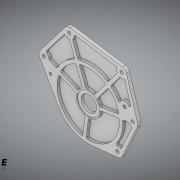
# Autodesk Inventor part: 後ろ脚内フレーム２
Saved by Autodesk Inventor 2020 (Build 240168000, 168)
## iProperties
Created: 2019-09-18
Part Number: 後ろ脚内フレーム２
Material: アルミニウム 2014-T4
Document SubType Name: Modeling
Designer: tanjihayato
Density: 2.8 g/cm^3
Appearance: サテン
Mass: 21.8846 g
Surface Area: 133.053 cm^2
Volume: 7.81591 cm^3
Author: tanjihayato
Autodesk Inventor part; units mm, degrees
ref_plane "YZ Plane" through (0, 0, 0) normal (1, 0, 0) x (0, 1, 0)
ref_plane "XZ Plane" through (0, 0, 0) normal (0, 1, 0) x (-1, 0, 0)
sketch "スケッチ1" plane through (0, 0, 0) normal (0, 0, 1) x (1, 0, 0)
  circle A0 centre (-21.6908, -16.4118) radius 19.1 construction
  circle A1 centre (-58.0056, -24.4791) radius 22.1 construction
  circle A2 centre (-105.5257, -16.4118) radius 30.1 construction
  circle A3 centre (-122.6945, 30.2622) radius 1.5
  circle A4 centre (-75.5257, 23.124) radius 1.5
  circle A5 centre (-65.5257, -10.4118) radius 1.5
  circle A6 centre (-145.5257, 0.5882) radius 1.5
  circle A7 centre (-105.5257, -16.4118) radius 7.025
  circle A8 centre (-21.6908, -16.4118) radius 1.5
  arc A9 (-17.8785, -18.8026) -> (-19.2493, -12.6317) centre (-21.6908, -16.4118) ccw
  arc A10 (-61.0009, -47.384) -> (-50.9717, -46.4821) centre (-58.0056, -24.4791) ccw
  circle A11 centre (-34.2292, -36.4056) radius 1.5
  circle A12 centre (-41.5152, -3.6073) radius 1.5
  arc A13 (-39.0737, 0.1727) -> (-41.3386, 0.8892) centre (-41.5152, -3.6073) ccw
  arc A14 (-32.8589, -40.6919) -> (-30.4168, -38.7963) centre (-34.2292, -36.4056) ccw
  circle A15 centre (-79.2726, -40.4563) radius 1.5
  arc A16 (-78.813, -44.9328) -> (-75.1806, -42.3286) centre (-79.2726, -40.4563) ccw
  line L0 (-17.8785, -18.8026) -> (-30.4168, -38.7963)
  line L1 (-32.8589, -40.6919) -> (-50.9717, -46.4821)
  line L2 (-19.2493, -12.6317) -> (-39.0737, 0.1727)
  arc A17 (-149.0922, 3.3323) -> (-149.4523, -1.6098) centre (-145.5257, 0.5882) ccw
  line L3 (-149.4523, -1.6098) -> (-132.6633, -31.6026)
  line L4 (-102.3494, -47.3492) -> (-78.813, -44.9328)
  line L5 (-61.0009, -47.384) -> (-79.8561, -44.9183)
  circle A18 centre (-72.8083, -2.3784) radius 1.5
  arc A19 (-72.6317, 2.1181) -> (-76.944, -4.1523) centre (-72.8083, -2.3784) ccw
  line L6 (-41.3386, 0.8892) -> (-72.6317, 2.1181)
  arc A20 (-61.4337, -12.2841) -> (-61.2133, -9.1259) centre (-65.5257, -10.4118) ccw
  line L7 (-61.4337, -12.2841) -> (-75.1806, -42.3286)
  arc A21 (-82.5911, -37.417) -> (-76.944, -4.1523) centre (-105.5257, -16.4118) ccw
  arc A22 (-132.6633, -31.6026) -> (-102.3494, -47.3492) centre (-105.5257, -16.4118) ccw
  arc A23 (-122.0212, 34.7115) -> (-126.261, 33.0062) centre (-122.6945, 30.2622) ccw
  arc A24 (-71.2133, 24.4099) -> (-74.8523, 27.5733) centre (-75.5257, 23.124) ccw
  line L8 (-126.261, 33.0062) -> (-149.0922, 3.3323)
  line L9 (-122.0212, 34.7115) -> (-74.8523, 27.5733)
  line L10 (-71.2133, 24.4099) -> (-61.2133, -9.1259)
  circle A25 centre (-58.0056, -24.4791) radius 1.5
  point P0 (0, 0)
  point P1 (0, 0)
  dimension "d0" = 14.05
  dimension "d1" = 3
  dimension "d2" = 3
  dimension "d3" = 1
  dimension "d4" = 3
  dimension "d5" = 3
  dimension "d6" = 3
  dimension "d7" = 3
  dimension "d8" = 3
  dimension "d9" = 3
  dimension "d10" = 9
  dimension "d11" = 3
  dimension "d12" = 3
  dimension "d13" = 9
  dimension "d14" = 31.1
  dimension "d15" = 31.1
  dimension "d16" = 9
  dimension "d17" = 9
  dimension "d18" = 3
  constraints: 30 tangent, 26 centre point, 24 point on circle, 22 end point, 9 coincident
  measures "d0" diameter of A7
  measures "d1" diameter of A8
  measures "d2" radial gap between concentric circles of A8 A9
  measures "d3" radial gap between concentric circles of A1 A10
  measures "d4" diameter of A11
  measures "d5" diameter of A12
  measures "d6" radial gap between concentric circles of A12 A13
  measures "d7" radial gap between concentric circles of A11 A14
  measures "d8" diameter of A15
  measures "d9" radial gap between concentric circles of A15 A16
  measures "d10" diameter of A17
  measures "d11" diameter of A18
  measures "d12" radial gap between concentric circles of A18 A19
  measures "d13" diameter of A20
  measures "d14" radius of A22
  measures "d15" radius of A21
  measures "d16" diameter of A23
  measures "d17" diameter of A24
  measures "d18" diameter of A25
extrude "押し出し1" add sketch "スケッチ1" along normal blind 3 contours L10 A20 L7 A16 L4 A22 L3 A17 L8 A23 L9 A24
sketch "スケッチ2" plane through (0, 0, 3) normal (0, 0, 1) x (1, 0, 0)
  circle A0 centre (-105.5257, -16.4118) radius 30.1 construction
  line L0 (-132.6633, -31.6026) -> (-149.4523, -1.6098) projected
  circle A1 centre (-139.5445, -10.0968) radius 4.5 construction
  line L1 (-149.4523, -1.6098) -> (-132.6633, -31.6026) projected
  circle A2 centre (-139.5445, -10.0968) radius 1.25
  point P0 (0, 0)
  dimension "d21" = 9
  dimension "d22" = 2.5
  constraints: 2 centre point, 2 tangent, 1 coincident
  measures "d21" diameter of A1
  measures "d22" diameter of A2
extrude "押し出し2" cut sketch "スケッチ2" against normal blind 10
sketch "スケッチ3" plane through (0, 0, 3) normal (0, 0, 1) x (1, 0, 0)
  circle A0 centre (-139.5445, -10.0968) radius 1.25 projected
  circle A1 centre (-105.5257, -16.4118) radius 7.025 projected
  circle A2 centre (-72.8083, -2.3784) radius 1.5 projected
  circle A3 centre (-79.2726, -40.4563) radius 1.5 projected
  circle A4 centre (-145.5257, 0.5882) radius 1.5 projected
  circle A5 centre (-65.5257, -10.4118) radius 1.5 projected
  circle A6 centre (-75.5257, 23.124) radius 1.5 projected
  circle A7 centre (-122.6945, 30.2622) radius 1.5 projected
  line L0 (-126.261, 33.0062) -> (-149.0922, 3.3323) projected
  arc A8 (-149.0922, 3.3323) -> (-149.4523, -1.6098) centre (-145.5257, 0.5882) ccw projected
  line L1 (-149.4523, -1.6098) -> (-132.6633, -31.6026) projected
  arc A9 (-132.6633, -31.6026) -> (-102.3494, -47.3492) centre (-105.5257, -16.4118) ccw projected
  line L2 (-102.3494, -47.3492) -> (-78.813, -44.9328) projected
  arc A10 (-78.813, -44.9328) -> (-75.1806, -42.3286) centre (-79.2726, -40.4563) ccw projected
  line L3 (-75.1806, -42.3286) -> (-61.4337, -12.2841) projected
  arc A11 (-61.4337, -12.2841) -> (-61.2133, -9.1259) centre (-65.5257, -10.4118) ccw projected
  line L4 (-61.2133, -9.1259) -> (-71.2133, 24.4099) projected
  arc A12 (-71.2133, 24.4099) -> (-74.8523, 27.5733) centre (-75.5257, 23.124) ccw projected
  line L5 (-74.8523, 27.5733) -> (-122.0212, 34.7115) projected
  arc A13 (-122.0212, 34.7115) -> (-126.261, 33.0062) centre (-122.6945, 30.2622) ccw projected
  line L6 (-118.2752, 31.1105) -> (-79.4961, 25.2419)
  arc A14 (-74.0882, 23.5526) -> (-75.3012, 24.6071) centre (-75.5257, 23.124) ccw
  line L7 (-72.8759, 19.4869) -> (-65.3006, -5.9174)
  arc A15 (-64.1617, -11.0359) -> (-64.0882, -9.9832) centre (-65.5257, -10.4118) ccw
  line L8 (-65.9269, -14.8939) -> (-76.1434, -37.2224)
  arc A16 (-79.1194, -41.9485) -> (-77.9086, -41.0804) centre (-79.2726, -40.4563) ccw
  line L9 (-83.3399, -42.3818) -> (-89.3988, -43.0038)
  arc A17 (-146.7145, 1.5029) -> (-146.8346, -0.1445) centre (-145.5257, 0.5882) ccw
  line L10 (-144.1274, 4.8654) -> (-126.4705, 27.8143)
  arc A18 (-122.47, 31.7453) -> (-123.8833, 31.1769) centre (-122.6945, 30.2622) ccw
  circle A19 centre (-72.8083, -2.3784) radius 4.5
  arc A20 (-76.1434, -37.2224) -> (-82.5911, -37.417) centre (-79.2726, -40.4563) ccw
  circle A21 centre (-105.5257, -16.4118) radius 10.025
  line L11 (-122.6945, 30.2622) -> (-105.5257, -16.4118) construction
  arc A22 (-121.2867, 30.78) -> (-124.1023, 29.7443) centre (-122.6945, 30.2622) ccw
  arc A23 (-106.9334, -16.9296) -> (-104.1179, -15.894) centre (-105.5257, -16.4118) ccw
  line L12 (-75.5257, 23.124) -> (-105.5257, -16.4118) construction
  arc A24 (-74.3307, 22.2173) -> (-76.7206, 24.0307) centre (-75.5257, 23.124) ccw
  arc A25 (-106.7206, -15.5051) -> (-104.3307, -17.3185) centre (-105.5257, -16.4118) ccw
  line L13 (-105.5257, -16.4118) -> (-65.5257, -10.4118) construction
  arc A26 (-105.7482, -14.9284) -> (-105.3032, -17.8952) centre (-105.5257, -16.4118) ccw
  arc A27 (-65.3032, -11.8952) -> (-65.7482, -8.9284) centre (-65.5257, -10.4118) ccw
  line L14 (-145.5257, 0.5882) -> (-105.5257, -16.4118) construction
  arc A28 (-144.939, 1.9687) -> (-146.1124, -0.7923) centre (-145.5257, 0.5882) ccw
  arc A29 (-106.1124, -17.7923) -> (-104.939, -15.0313) centre (-105.5257, -16.4118) ccw
  line L15 (-105.5257, -16.4118) -> (-109.0706, -44.2873) construction
  arc A30 (-104.0377, -16.601) -> (-107.0137, -16.2226) centre (-105.5257, -16.4118) ccw
  arc A31 (-110.298, -45.1495) -> (-107.5826, -44.4765) centre (-109.0706, -44.2873) ccw
  arc A32 (-144.7622, -3.8466) -> (-142.2077, -2.4518) centre (-145.5257, 0.5882) ccw
  arc A33 (-141.0343, 0.3092) -> (-144.1274, 4.8654) centre (-145.5257, 0.5882) ccw
  line L16 (-136.5549, -18.5085) -> (-138.9111, -14.2994)
  line L17 (-142.7957, -7.3597) -> (-144.7622, -3.8466)
  arc A34 (-138.9111, -14.2994) -> (-136.4376, -12.9968) centre (-139.5445, -10.0968) ccw
  arc A35 (-135.6038, -8.5052) -> (-142.7957, -7.3597) centre (-139.5445, -10.0968) ccw
  arc A36 (-136.4376, -12.9968) -> (-136.5549, -18.5085) centre (-105.5257, -16.4118) ccw
  arc A37 (-130.0455, -30.1373) -> (-110.5535, -44.0583) centre (-105.5257, -16.4118) ccw
  arc A38 (-107.5775, -44.4368) -> (-102.6558, -44.3649) centre (-105.5257, -16.4118) ccw
  arc A39 (-132.6633, -31.6026) -> (-102.3494, -47.3492) centre (-105.5257, -16.4118) ccw
  arc A40 (-65.3006, -5.9174) -> (-69.9439, -9.5578) centre (-65.5257, -10.4118) ccw
  arc A41 (-69.4989, -12.5246) -> (-65.9269, -14.8939) centre (-65.5257, -10.4118) ccw
  line L18 (-74.583, -13.2872) -> (-69.4989, -12.5246)
  line L19 (-69.9439, -9.5578) -> (-75.0281, -10.3204)
  line L20 (-85.5533, 7.4275) -> (-76.8953, 18.8375)
  line L21 (-79.2852, 20.6509) -> (-87.9431, 9.241)
  line L22 (-114.842, 13.26) -> (-119.822, 26.7982)
  line L23 (-122.6376, 25.7625) -> (-117.6576, 12.2243)
  line L24 (-133.5279, -2.881) -> (-141.0343, 0.3092)
  line L25 (-142.2077, -2.4518) -> (-134.7014, -5.642)
  arc A42 (-131.9368, -6.8169) -> (-110.5535, -44.0583) centre (-105.5257, -16.4118) ccw
  arc A43 (-134.7014, -5.642) -> (-135.6038, -8.5052) centre (-105.5257, -16.4118) ccw
  arc A44 (-116.6206, 9.4051) -> (-130.7634, -4.0559) centre (-105.5257, -16.4118) ccw
  arc A45 (-117.6576, 12.2243) -> (-133.5279, -2.881) centre (-105.5257, -16.4118) ccw
  arc A46 (-126.4705, 27.8143) -> (-122.6376, 25.7625) centre (-122.6945, 30.2622) ccw
  arc A47 (-119.822, 26.7982) -> (-118.2752, 31.1105) centre (-122.6945, 30.2622) ccw
  arc A48 (-89.7589, 6.848) -> (-113.805, 10.4408) centre (-105.5257, -16.4118) ccw
  arc A49 (-87.9431, 9.241) -> (-114.842, 13.26) centre (-105.5257, -16.4118) ccw
  arc A50 (-79.4961, 25.2419) -> (-79.2852, 20.6509) centre (-75.5257, 23.124) ccw
  arc A51 (-76.8953, 18.8375) -> (-72.8759, 19.4869) centre (-75.5257, 23.124) ccw
  line L26 (-105.3032, -17.8952) -> (-98.5161, -16.8771)
  line L27 (-95.5007, -16.4248) -> (-77.5537, -13.7328)
  line L28 (-77.9987, -10.766) -> (-95.9457, -13.458)
  line L29 (-98.9611, -13.9103) -> (-105.7482, -14.9284)
  line L30 (-104.3307, -17.3185) -> (-100.1822, -11.8513)
  line L31 (-98.339, -9.4223) -> (-87.3691, 5.0346)
  line L32 (-89.7589, 6.848) -> (-100.7289, -7.6089)
  line L33 (-102.5721, -10.0379) -> (-106.7206, -15.5051)
  line L34 (-104.1179, -15.894) -> (-106.4872, -9.4529)
  line L35 (-107.5399, -6.5912) -> (-113.805, 10.4408)
  line L36 (-116.6206, 9.4051) -> (-110.3554, -7.6269)
  line L37 (-109.3028, -10.4886) -> (-106.9334, -16.9296)
  line L38 (-104.939, -15.0313) -> (-111.2552, -12.3469)
  line L39 (-114.0614, -11.1543) -> (-130.7634, -4.0559)
  line L40 (-131.9368, -6.8169) -> (-115.2348, -13.9153)
  line L41 (-112.4286, -15.1079) -> (-106.1124, -17.7923)
  line L42 (-107.0137, -16.2226) -> (-107.8795, -23.0307)
  line L43 (-108.2641, -26.0555) -> (-110.5535, -44.0583)
  line L44 (-107.5775, -44.4368) -> (-105.2881, -26.434)
  line L45 (-104.9034, -23.4092) -> (-104.0377, -16.601)
  arc A52 (-82.5911, -37.417) -> (-74.583, -13.2872) centre (-105.5257, -16.4118) ccw
  arc A53 (-75.0281, -10.3204) -> (-85.5533, 7.4275) centre (-105.5257, -16.4118) ccw
  arc A54 (-107.5775, -44.4368) -> (-77.5537, -13.7328) centre (-105.5257, -16.4118) ccw
  arc A55 (-77.9987, -10.766) -> (-87.3691, 5.0346) centre (-105.5257, -16.4118) ccw
  point P0 (0, 0)
  point P1 (-114.1101, 6.9252)
  point P2 (-90.5257, 3.3561)
  point P3 (-85.5257, -13.4118)
  point P4 (-125.5257, -7.9118)
  point P5 (-107.2981, -30.3496)
  dimension "d28" = 3
  dimension "d25" = 3
  dimension "d27" = 3
  dimension "d30" = 3
  dimension "d31" = 3
  dimension "d32" = 3
  dimension "d33" = 3
  dimension "d38" = 3
  dimension "d39" = 3
  dimension "d40" = 105.778
  dimension "d41" = 105.778
  constraints: 92 end point, 80 point on circle, 56 tangent, 41 centre point, 40 parallel, 5 midpoint, 1 coincident, 1 concentric, 1 point on line, 23 other
  measures "d25" distance between parallel lines of L5 L6
  measures "d27" radial gap between concentric circles of A2 A19
  measures "d30" diameter of A23
  measures "d31" diameter of A25
  measures "d32" diameter of A27
  measures "d33" radial gap between concentric circles of A20 A3
  measures "d38" diameter of A29
  measures "d39" diameter of A31
  measures "d40" angle of L15 L13
  measures "d41" angle of L14 L15
extrude "押し出し3" cut sketch "スケッチ3" against normal blind 2.5 contours L6 A50 L21 A49 L22 A47 | L7 A40 L19 A53 L20 A51 | L8 A20 A52 L18 A41 | L10 A46 L23 A45 L24 A33 | A21 L31 A55 L28 | L27 A54 A38 L44 A21 | A21 L35 A48 L32 | L43 A37 A42 L40 A21 | A21 L39 A44 L36
sketch "スケッチ4" plane through (0, 0, 3) normal (0, 0, 1) x (1, 0, 0)
  arc A0 (-115.2348, -13.9153) -> (-108.2641, -26.0555) centre (-105.5257, -16.4118) ccw projected
  line L0 (-108.2641, -26.0555) -> (-110.5535, -44.0583) projected
  arc A1 (-131.9368, -6.8169) -> (-110.5535, -44.0583) centre (-105.5257, -16.4118) ccw projected
  line L1 (-131.9368, -6.8169) -> (-115.2348, -13.9153) projected
  arc A2 (-119.822, 26.7982) -> (-118.2752, 31.1105) centre (-122.6945, 30.2622) ccw projected
  line L2 (-118.2752, 31.1105) -> (-79.4961, 25.2419) projected
  arc A3 (-79.4961, 25.2419) -> (-79.2852, 20.6509) centre (-75.5257, 23.124) ccw projected
  line L3 (-79.2852, 20.6509) -> (-87.9431, 9.241) projected
  arc A4 (-87.9431, 9.241) -> (-114.842, 13.26) centre (-105.5257, -16.4118) ccw projected
  line L4 (-114.842, 13.26) -> (-119.822, 26.7982) projected
  arc A5 (-76.8953, 18.8375) -> (-72.8759, 19.4869) centre (-75.5257, 23.124) ccw projected
  line L5 (-72.8759, 19.4869) -> (-65.3006, -5.9174) projected
  arc A6 (-65.3006, -5.9174) -> (-69.9439, -9.5578) centre (-65.5257, -10.4118) ccw projected
  line L6 (-69.9439, -9.5578) -> (-75.0281, -10.3204) projected
  arc A7 (-75.0281, -10.3204) -> (-76.944, -4.1523) centre (-105.5257, -16.4118) ccw projected
  arc A8 (-76.944, -4.1523) -> (-85.5533, 7.4275) centre (-105.5257, -16.4118) ccw projected
  line L7 (-85.5533, 7.4275) -> (-76.8953, 18.8375) projected
  line L8 (-114.0614, -11.1543) -> (-130.7634, -4.0559) projected
  arc A9 (-116.6206, 9.4051) -> (-130.7634, -4.0559) centre (-105.5257, -16.4118) ccw projected
  line L9 (-116.6206, 9.4051) -> (-110.3554, -7.6269) projected
  arc A10 (-110.3554, -7.6269) -> (-114.0614, -11.1543) centre (-105.5257, -16.4118) ccw projected
  line L10 (-65.9269, -14.8939) -> (-76.1434, -37.2224) projected
  arc A11 (-76.1434, -37.2224) -> (-82.5911, -37.417) centre (-79.2726, -40.4563) ccw projected
  arc A12 (-82.5911, -37.417) -> (-74.583, -13.2872) centre (-105.5257, -16.4118) ccw projected
  line L11 (-74.583, -13.2872) -> (-69.4989, -12.5246) projected
  arc A13 (-69.4989, -12.5246) -> (-65.9269, -14.8939) centre (-65.5257, -10.4118) ccw projected
  line L12 (-98.339, -9.4223) -> (-87.3691, 5.0346) projected
  arc A14 (-77.9987, -10.766) -> (-87.3691, 5.0346) centre (-105.5257, -16.4118) ccw projected
  line L13 (-77.9987, -10.766) -> (-95.9457, -13.458) projected
  arc A15 (-95.9457, -13.458) -> (-98.339, -9.4223) centre (-105.5257, -16.4118) ccw projected
  arc A16 (-100.7289, -7.6089) -> (-107.5399, -6.5912) centre (-105.5257, -16.4118) ccw projected
  line L14 (-107.5399, -6.5912) -> (-113.805, 10.4408) projected
  arc A17 (-89.7589, 6.848) -> (-113.805, 10.4408) centre (-105.5257, -16.4118) ccw projected
  line L15 (-89.7589, 6.848) -> (-100.7289, -7.6089) projected
  line L16 (-133.5279, -2.881) -> (-141.0343, 0.3092) projected
  arc A18 (-141.0343, 0.3092) -> (-144.1274, 4.8654) centre (-145.5257, 0.5882) ccw projected
  line L17 (-144.1274, 4.8654) -> (-126.4705, 27.8143) projected
  arc A19 (-126.4705, 27.8143) -> (-122.6376, 25.7625) centre (-122.6945, 30.2622) ccw projected
  line L18 (-122.6376, 25.7625) -> (-117.6576, 12.2243) projected
  arc A20 (-117.6576, 12.2243) -> (-133.5279, -2.881) centre (-105.5257, -16.4118) ccw projected
  line L19 (-95.5007, -16.4248) -> (-77.5537, -13.7328) projected
  arc A21 (-107.5775, -44.4368) -> (-77.5537, -13.7328) centre (-105.5257, -16.4118) ccw projected
  line L20 (-107.5775, -44.4368) -> (-105.2881, -26.434) projected
  arc A22 (-105.2881, -26.434) -> (-95.5007, -16.4248) centre (-105.5257, -16.4118) ccw projected
  circle A23 centre (-139.5445, -10.0968) radius 1.25 projected
  circle A24 centre (-105.5257, -16.4118) radius 7.025 projected
  circle A25 centre (-79.2726, -40.4563) radius 1.5 projected
  circle A26 centre (-145.5257, 0.5882) radius 1.5 projected
  circle A27 centre (-65.5257, -10.4118) radius 1.5 projected
  circle A28 centre (-75.5257, 23.124) radius 1.5 projected
  circle A29 centre (-122.6945, 30.2622) radius 1.5 projected
  line L21 (-126.261, 33.0062) -> (-149.0922, 3.3323) projected
  arc A30 (-149.0922, 3.3323) -> (-149.4523, -1.6098) centre (-145.5257, 0.5882) ccw projected
  line L22 (-149.4523, -1.6098) -> (-132.6633, -31.6026) projected
  arc A31 (-132.6633, -31.6026) -> (-102.3494, -47.3492) centre (-105.5257, -16.4118) ccw projected
  line L23 (-102.3494, -47.3492) -> (-78.813, -44.9328) projected
  arc A32 (-78.813, -44.9328) -> (-75.1806, -42.3286) centre (-79.2726, -40.4563) ccw projected
  line L24 (-75.1806, -42.3286) -> (-61.4337, -12.2841) projected
  arc A33 (-61.4337, -12.2841) -> (-61.2133, -9.1259) centre (-65.5257, -10.4118) ccw projected
  line L25 (-61.2133, -9.1259) -> (-71.2133, 24.4099) projected
  arc A34 (-71.2133, 24.4099) -> (-74.8523, 27.5733) centre (-75.5257, 23.124) ccw projected
  line L26 (-74.8523, 27.5733) -> (-122.0212, 34.7115) projected
  arc A35 (-122.0212, 34.7115) -> (-126.261, 33.0062) centre (-122.6945, 30.2622) ccw projected
  circle A36 centre (-105.5257, -16.4118) radius 11
  circle A37 centre (-105.5257, -16.4118) radius 10
  point P0 (0, 0)
  dimension "d44" = 22
  dimension "d45" = 20
  constraints: 2 centre point, 2 coincident
  measures "d44" diameter of A36
  measures "d45" diameter of A37
extrude "押し出し4" add sketch "スケッチ4" against normal blind 2.5 contours L1 A36 L8 A10 L9 L14 A16 L15 L12 A15 L13 L19 A22 L20 L0 A0 | A0 L0 A36 L1 | A36 L9 A10 L8 | L20 A22 L19 A36 | A36 L15 A16 L14 | L13 A15 L12 A36
extrude "押し出し5" cut sketch "スケッチ4" against normal blind 0.5 contours A37
sketch "スケッチ5" plane through (-72.8083, -2.3784, 3) normal (0, 0, 1) x (1, 0, 0)
  arc A0 (3.6342, 2.6538) -> (-4.1186, 1.813) centre (0, 0) ccw
  circle A1 centre (0, 0) radius 1.5 projected
  circle A2 centre (-32.7173, -14.0334) radius 10 projected
  line L0 (-53.4527, 35.3847) -> (-76.2838, 5.7107) projected
  arc A3 (-76.2838, 5.7107) -> (-76.644, 0.7686) centre (-72.7173, 2.9666) ccw projected
  line L1 (-76.644, 0.7686) -> (-59.8549, -29.2242) projected
  arc A4 (-59.8549, -29.2242) -> (-29.5411, -44.9708) centre (-32.7173, -14.0334) ccw projected
  line L2 (-29.5411, -44.9708) -> (-6.0047, -42.5544) projected
  arc A5 (-6.0047, -42.5544) -> (-2.3723, -39.9502) centre (-6.4643, -38.0779) ccw projected
  line L3 (-2.3723, -39.9502) -> (11.3747, -9.9057) projected
  arc A6 (11.3747, -9.9057) -> (11.595, -6.7475) centre (7.2827, -8.0334) ccw projected
  line L4 (11.595, -6.7475) -> (1.595, 26.7883) projected
  arc A7 (1.595, 26.7883) -> (-2.044, 29.9517) centre (-2.7173, 25.5024) ccw projected
  line L5 (-2.044, 29.9517) -> (-49.2128, 37.0899) projected
  arc A8 (-49.2128, 37.0899) -> (-53.4527, 35.3847) centre (-49.8862, 32.6406) ccw projected
  circle A9 centre (-49.8862, 32.6406) radius 1.5 projected
  circle A10 centre (-2.7173, 25.5024) radius 1.5 projected
  circle A11 centre (7.2827, -8.0334) radius 1.5 projected
  circle A12 centre (-72.7173, 2.9666) radius 1.5 projected
  circle A13 centre (-6.4643, -38.0779) radius 1.5 projected
  circle A14 centre (-66.7362, -7.7184) radius 1.25 projected
  line L6 (-60.7196, -0.5026) -> (-68.226, 2.6876) projected
  arc A15 (-68.226, 2.6876) -> (-71.319, 7.2438) centre (-72.7173, 2.9666) ccw projected
  line L7 (-71.319, 7.2438) -> (-53.6621, 30.1927) projected
  arc A16 (-53.6621, 30.1927) -> (-49.8292, 28.1409) centre (-49.8862, 32.6406) ccw projected
  line L8 (-49.8292, 28.1409) -> (-44.8493, 14.6027) projected
  arc A17 (-44.8493, 14.6027) -> (-60.7196, -0.5026) centre (-32.7173, -14.0334) ccw projected
  line L9 (6.8814, -12.5155) -> (-3.3351, -34.844) projected
  arc A18 (-3.3351, -34.844) -> (-9.7828, -35.0386) centre (-6.4643, -38.0779) ccw projected
  arc A19 (-9.7828, -35.0386) -> (-1.7747, -10.9088) centre (-32.7173, -14.0334) ccw projected
  line L10 (-1.7747, -10.9088) -> (3.3095, -10.1461) projected
  arc A20 (3.3095, -10.1461) -> (6.8814, -12.5155) centre (7.2827, -8.0334) ccw projected
  arc A21 (-4.087, 21.2159) -> (-0.0675, 21.8653) centre (-2.7173, 25.5024) ccw projected
  line L11 (-0.0675, 21.8653) -> (7.5078, -3.539) projected
  arc A22 (7.5078, -3.539) -> (2.8645, -7.1793) centre (7.2827, -8.0334) ccw projected
  line L12 (2.8645, -7.1793) -> (-2.2197, -7.942) projected
  arc A23 (-2.2197, -7.942) -> (-4.1356, -1.7739) centre (-32.7173, -14.0334) ccw projected
  arc A24 (-4.1356, -1.7739) -> (-12.7449, 9.8059) centre (-32.7173, -14.0334) ccw projected
  line L13 (-12.7449, 9.8059) -> (-4.087, 21.2159) projected
  arc A25 (-47.0137, 29.1766) -> (-45.4668, 33.4889) centre (-49.8862, 32.6406) ccw projected
  line L14 (-45.4668, 33.4889) -> (-6.6878, 27.6203) projected
  arc A26 (-6.6878, 27.6203) -> (-6.4769, 23.0293) centre (-2.7173, 25.5024) ccw projected
  line L15 (-6.4769, 23.0293) -> (-15.1348, 11.6194) projected
  arc A27 (-15.1348, 11.6194) -> (-42.0337, 15.6384) centre (-32.7173, -14.0334) ccw projected
  line L16 (-42.0337, 15.6384) -> (-47.0137, 29.1766) projected
  arc A28 (-22.1632, -10.9335) -> (-24.9352, -6.2591) centre (-32.7173, -14.0334) ccw projected
  line L17 (-24.9352, -6.2591) -> (-14.5607, 7.413) projected
  arc A29 (-5.1904, -8.3876) -> (-14.5607, 7.413) centre (-32.7173, -14.0334) ccw projected
  line L18 (-5.1904, -8.3876) -> (-22.1632, -10.9335) projected
  line L19 (-35.0716, -3.2883) -> (-40.9967, 12.8192) projected
  arc A30 (-16.9506, 9.2264) -> (-40.9967, 12.8192) centre (-32.7173, -14.0334) ccw projected
  line L20 (-16.9506, 9.2264) -> (-27.3251, -4.4457) projected
  arc A31 (-27.3251, -4.4457) -> (-35.0716, -3.2883) centre (-32.7173, -14.0334) ccw projected
  arc A32 (-32.604, -25.0328) -> (-21.7181, -13.9003) centre (-32.7173, -14.0334) ccw projected
  line L21 (-21.7181, -13.9003) -> (-4.7453, -11.3544) projected
  arc A33 (-34.7692, -42.0584) -> (-4.7453, -11.3544) centre (-32.7173, -14.0334) ccw projected
  line L22 (-34.7692, -42.0584) -> (-32.604, -25.0328) projected
  line L23 (-42.1597, -8.3905) -> (-57.9551, -1.6775) projected
  arc A34 (-43.8122, 11.7835) -> (-57.9551, -1.6775) centre (-32.7173, -14.0334) ccw projected
  line L24 (-43.8122, 11.7835) -> (-37.8872, -4.324) projected
  arc A35 (-37.8872, -4.324) -> (-42.1597, -8.3905) centre (-32.7173, -14.0334) ccw projected
  line L25 (-35.5801, -24.6543) -> (-37.7452, -41.6799) projected
  arc A36 (-59.1285, -4.4385) -> (-37.7452, -41.6799) centre (-32.7173, -14.0334) ccw projected
  line L26 (-59.1285, -4.4385) -> (-43.3331, -11.1515) projected
  arc A37 (-43.3331, -11.1515) -> (-35.5801, -24.6543) centre (-32.7173, -14.0334) ccw projected
  arc A38 (-5.8963, 1.7096) -> (-4.1186, 1.813) centre (-5.0339, 2.2158) ccw
  arc A39 (3.6342, 2.6538) -> (5.4001, 3.5293) centre (4.4418, 3.2436) ccw
  line L27 (-0.0675, 21.8653) -> (7.5078, -3.539) projected
  circle A40 centre (0, 0) radius 4.5 projected
  point P0 (72.8083, 2.3784)
  dimension "d50" = 2
  dimension "d51" = 2
  constraints: 10 point on circle, 4 centre point, 4 tangent, 1 point on line
  measures "d50" diameter of A38
  measures "d51" diameter of A39
extrude "押し出し6" add sketch "スケッチ5" against normal blind 3 contours A39 L11 A22 L12 A23 A40 | A40 A24 A38
fillet "フィレット1" radius 1 40 edges at (-144.1274, 4.8654, 1.75) (-141.0343, 0.3092, 1.75) (-133.5279, -2.881, 1.75) (-130.7634, -4.0559, 1.75) (-131.9368, -6.8169, 1.75) (-116.1415, -13.5299, 1.75) (-114.968, -10.7689, 1.75) (-110.6955, -6.7024, 1.75) (-107.8799, -5.6667, 1.75) (-116.6206, 9.4051, 1.75) (-117.6576, 12.2243, 1.75) (-114.842, 13.26, 1.75) (-113.805, 10.4408, 1.75) (-100.1334, -6.8241, 1.75) (-108.3884, -27.0328, 1.75) (-105.4124, -27.4112, 1.75) (-110.5535, -44.0583, 1.75) (-107.5775, -44.4368, 1.75) (-94.5265, -16.2787, 1.75) (-94.9715, -13.3119, 1.75) (-97.7436, -8.6376, 1.75) (-77.5537, -13.7328, 1.75) (-82.5911, -37.417, 1.75) (-76.1434, -37.2224, 1.75) (-65.9269, -14.8939, 1.75) (-69.4989, -12.5246, 1.75) (-74.583, -13.2872, 1.75) (-77.9987, -10.766, 1.75) (-87.3691, 5.0346, 1.75) (-89.7589, 6.848, 1.75) (-85.5533, 7.4275, 1.75) (-87.9431, 9.241, 1.75) (-72.8759, 19.4869, 1.75) (-76.8953, 18.8375, 1.75) (-79.2852, 20.6509, 1.75) (-79.4961, 25.2419, 1.75) (-119.822, 26.7982, 1.75) (-118.2752, 31.1105, 1.75) (-122.6376, 25.7625, 1.75) (-126.4705, 27.8143, 1.75)
sketch "スケッチ6" plane through (0, 0, 3) normal (0, 0, 1) x (1, 0, 0)
  circle A0 centre (-72.8083, -2.3784) radius 1.5 projected
  circle A1 centre (-105.5257, -16.4118) radius 10 projected
  line L0 (-126.261, 33.0062) -> (-149.0922, 3.3323) projected
  arc A2 (-149.0922, 3.3323) -> (-149.4523, -1.6098) centre (-145.5257, 0.5882) ccw projected
  line L1 (-149.4523, -1.6098) -> (-132.6633, -31.6026) projected
  arc A3 (-132.6633, -31.6026) -> (-102.3494, -47.3492) centre (-105.5257, -16.4118) ccw projected
  line L2 (-102.3494, -47.3492) -> (-78.813, -44.9328) projected
  arc A4 (-78.813, -44.9328) -> (-75.1806, -42.3286) centre (-79.2726, -40.4563) ccw projected
  line L3 (-75.1806, -42.3286) -> (-61.4337, -12.2841) projected
  arc A5 (-61.4337, -12.2841) -> (-61.2133, -9.1259) centre (-65.5257, -10.4118) ccw projected
  line L4 (-61.2133, -9.1259) -> (-71.2133, 24.4099) projected
  arc A6 (-71.2133, 24.4099) -> (-74.8523, 27.5733) centre (-75.5257, 23.124) ccw projected
  line L5 (-74.8523, 27.5733) -> (-122.0212, 34.7115) projected
  arc A7 (-122.0212, 34.7115) -> (-126.261, 33.0062) centre (-122.6945, 30.2622) ccw projected
  circle A8 centre (-122.6945, 30.2622) radius 1.5 projected
  circle A9 centre (-75.5257, 23.124) radius 1.5 projected
  circle A10 centre (-65.5257, -10.4118) radius 1.5 projected
  circle A11 centre (-145.5257, 0.5882) radius 1.5 projected
  circle A12 centre (-79.2726, -40.4563) radius 1.5 projected
  circle A13 centre (-139.5445, -10.0968) radius 1.25 projected
  line L6 (-134.3918, -2.5138) -> (-140.4303, 0.0525) projected
  arc A14 (-141.0367, 0.9029) -> (-140.4303, 0.0525) centre (-140.0391, 0.9728) ccw projected
  arc A15 (-141.0367, 0.9029) -> (-143.1172, 4.3894) centre (-145.5257, 0.5882) ccw projected
  arc A16 (-143.3745, 5.8439) -> (-143.1172, 4.3894) centre (-142.582, 5.2341) ccw projected
  line L7 (-143.3745, 5.8439) -> (-127.2233, 26.8358) projected
  arc A17 (-125.7514, 26.9599) -> (-127.2233, 26.8358) centre (-126.4308, 26.226) ccw projected
  arc A18 (-125.7514, 26.9599) -> (-123.2304, 25.7942) centre (-122.6945, 30.2622) ccw projected
  arc A19 (-122.411, 25.1465) -> (-123.2304, 25.7942) centre (-123.3495, 24.8013) ccw projected
  line L8 (-122.411, 25.1465) -> (-117.9817, 13.1053) projected
  arc A20 (-118.5029, 11.8513) -> (-117.9817, 13.1053) centre (-118.9202, 12.7601) ccw projected
  arc A21 (-118.5029, 11.8513) -> (-133.1136, -2.0551) centre (-105.5257, -16.4118) ccw projected
  arc A22 (-134.3918, -2.5138) -> (-133.1136, -2.0551) centre (-134.0007, -1.5935) ccw projected
  line L9 (-66.4406, -16.0165) -> (-75.6297, -36.0998) projected
  arc A23 (-77.0361, -36.5515) -> (-75.6297, -36.0998) centre (-76.5391, -35.6837) ccw projected
  arc A24 (-77.0361, -36.5515) -> (-79.315, -35.9565) centre (-79.2726, -40.4563) ccw projected
  arc A25 (-80.1407, -34.3788) -> (-79.315, -35.9565) centre (-79.3245, -34.9565) ccw projected
  arc A26 (-80.1407, -34.3788) -> (-74.5039, -14.2077) centre (-105.5257, -16.4118) ccw projected
  arc A27 (-73.6547, -13.1479) -> (-74.5039, -14.2077) centre (-73.5064, -14.1369) ccw projected
  line L10 (-73.6547, -13.1479) -> (-70.1479, -12.6219) projected
  arc A28 (-69.1862, -13.0292) -> (-70.1479, -12.6219) centre (-69.9996, -13.6109) ccw projected
  arc A29 (-69.1862, -13.0292) -> (-67.0182, -14.6571) centre (-65.5257, -10.4118) ccw projected
  arc A30 (-66.4406, -16.0165) -> (-67.0182, -14.6571) centre (-67.3499, -15.6005) ccw projected
  arc A31 (-69.1742, 0.2754) -> (-67.4083, 1.1509) centre (-68.3666, 0.8652) ccw projected
  arc A32 (-69.1742, 0.2754) -> (-76.927, -0.5655) centre (-72.8083, -2.3784) ccw projected
  arc A33 (-78.7046, -0.6688) -> (-76.927, -0.5655) centre (-77.8422, -0.1626) ccw projected
  arc A34 (-78.7046, -0.6688) -> (-84.8539, 6.8237) centre (-105.5257, -16.4118) ccw projected
  arc A35 (-84.9859, 8.1753) -> (-84.8539, 6.8237) centre (-84.1892, 7.5708) ccw projected
  line L11 (-84.9859, 8.1753) -> (-77.2921, 18.3146) projected
  arc A36 (-76.3191, 18.6945) -> (-77.2921, 18.3146) centre (-76.4955, 17.7101) ccw projected
  arc A37 (-76.3191, 18.6945) -> (-73.8531, 18.9464) centre (-75.5257, 23.124) ccw projected
  arc A38 (-72.5231, 18.3038) -> (-73.8531, 18.9464) centre (-73.4814, 18.018) ccw projected
  line L12 (-72.5231, 18.3038) -> (-67.4083, 1.1509) projected
  arc A39 (-119.391, 27.2065) -> (-118.2024, 29.9961) centre (-122.6945, 30.2622) ccw projected
  arc A40 (-117.0545, 30.9257) -> (-118.2024, 29.9961) centre (-117.2041, 29.937) ccw projected
  line L13 (-117.0545, 30.9257) -> (-80.7168, 25.4266) projected
  arc A41 (-79.8954, 24.199) -> (-80.7168, 25.4266) centre (-80.8664, 24.4379) ccw projected
  arc A42 (-79.8954, 24.199) -> (-79.578, 21.1674) centre (-75.5257, 23.124) ccw projected
  arc A43 (-79.6819, 20.1281) -> (-79.578, 21.1674) centre (-80.4786, 20.7325) ccw projected
  line L14 (-79.6819, 20.1281) -> (-87.3757, 9.9888) projected
  arc A44 (-88.7129, 9.752) -> (-87.3757, 9.9888) centre (-88.1723, 10.5932) ccw projected
  arc A45 (-88.7129, 9.752) -> (-113.9565, 13.5236) centre (-105.5257, -16.4118) ccw projected
  arc A46 (-115.1661, 14.141) -> (-113.9565, 13.5236) centre (-114.2276, 14.4862) ccw projected
  line L15 (-115.1661, 14.141) -> (-119.5954, 26.1822) projected
  arc A47 (-119.391, 27.2065) -> (-119.5954, 26.1822) centre (-118.6569, 26.5275) ccw projected
  line L16 (-97.2361, -7.9688) -> (-88.0192, 4.1778) projected
  arc A48 (-86.5472, 4.3108) -> (-88.0192, 4.1778) centre (-87.2226, 3.5733) ccw projected
  arc A49 (-78.2396, -9.6976) -> (-86.5472, 4.3108) centre (-105.5257, -16.4118) ccw projected
  arc A50 (-79.0623, -10.9255) -> (-78.2396, -9.6976) centre (-79.2106, -9.9366) ccw projected
  line L17 (-79.0623, -10.9255) -> (-94.1413, -13.1874) projected
  arc A51 (-95.226, -12.5495) -> (-94.1413, -13.1874) centre (-94.2897, -12.1984) ccw projected
  arc A52 (-95.226, -12.5495) -> (-97.1967, -9.2265) centre (-105.5257, -16.4118) ccw projected
  arc A53 (-97.2361, -7.9688) -> (-97.1967, -9.2265) centre (-96.4395, -8.5733) ccw projected
  line L18 (-108.1697, -4.8789) -> (-113.4337, 9.4314) projected
  arc A54 (-112.7524, 10.743) -> (-113.4337, 9.4314) centre (-112.4952, 9.7767) ccw projected
  arc A55 (-90.6772, 7.4447) -> (-112.7524, 10.743) centre (-105.5257, -16.4118) ccw projected
  arc A56 (-90.409, 5.9913) -> (-90.6772, 7.4447) centre (-91.2057, 6.5957) ccw projected
  line L19 (-90.409, 5.9913) -> (-99.626, -6.1554) projected
  arc A57 (-100.8479, -6.456) -> (-99.626, -6.1554) centre (-100.4226, -5.5509) ccw projected
  arc A58 (-100.8479, -6.456) -> (-107.0891, -5.5235) centre (-105.5257, -16.4118) ccw projected
  arc A59 (-108.1697, -4.8789) -> (-107.0891, -5.5235) centre (-107.2312, -4.5336) ccw projected
  line L20 (-93.6963, -16.1542) -> (-78.6173, -13.8923) projected
  arc A60 (-77.4705, -14.8248) -> (-78.6173, -13.8923) centre (-78.4689, -14.8813) ccw projected
  arc A61 (-106.4839, -44.4955) -> (-77.4705, -14.8248) centre (-105.5257, -16.4118) ccw projected
  arc A62 (-107.4418, -43.3699) -> (-106.4839, -44.4955) centre (-106.4498, -43.496) ccw projected
  line L21 (-107.4418, -43.3699) -> (-105.5183, -28.244) projected
  arc A63 (-104.6095, -27.3736) -> (-105.5183, -28.244) centre (-104.5263, -28.3701) ccw projected
  arc A64 (-104.6095, -27.3736) -> (-94.5461, -17.0822) centre (-105.5257, -16.4118) ccw projected
  arc A65 (-93.6963, -16.1542) -> (-94.5461, -17.0822) centre (-93.548, -17.1431) ccw projected
  line L22 (-115.7406, -10.4406) -> (-129.7736, -4.4766) projected
  arc A66 (-130.2628, -3.0819) -> (-129.7736, -4.4766) centre (-129.3824, -3.5563) ccw projected
  arc A67 (-117.6181, 8.9532) -> (-130.2628, -3.0819) centre (-105.5257, -16.4118) ccw projected
  arc A68 (-116.2493, 8.3957) -> (-117.6181, 8.9532) centre (-117.1878, 8.0505) ccw projected
  line L23 (-116.2493, 8.3957) -> (-110.9853, -5.9145) projected
  arc A69 (-111.3906, -7.1058) -> (-110.9853, -5.9145) centre (-111.9238, -6.2598) ccw projected
  arc A70 (-111.3906, -7.1058) -> (-114.5308, -10.0946) centre (-105.5257, -16.4118) ccw projected
  arc A71 (-115.7406, -10.4406) -> (-114.5308, -10.0946) centre (-115.3495, -9.5203) ccw projected
  line L24 (-108.4943, -27.8655) -> (-110.4179, -42.9914) projected
  arc A72 (-111.627, -43.8414) -> (-110.4179, -42.9914) centre (-111.4099, -42.8653) ccw projected
  arc A73 (-132.2906, -7.8533) -> (-111.627, -43.8414) centre (-105.5257, -16.4118) ccw projected
  arc A74 (-130.947, -7.2376) -> (-132.2906, -7.8533) centre (-131.3381, -8.1579) ccw projected
  line L25 (-130.947, -7.2376) -> (-116.914, -13.2016) projected
  arc A75 (-116.3235, -14.3128) -> (-116.914, -13.2016) centre (-117.3052, -14.1219) ccw projected
  arc A76 (-116.3235, -14.3128) -> (-109.1563, -26.7954) centre (-105.5257, -16.4118) ccw projected
  arc A77 (-108.4943, -27.8655) -> (-109.1563, -26.7954) centre (-109.4863, -27.7393) ccw projected
  circle A78 centre (-105.5257, -16.4118) radius 7.025 projected
  point P0 (0, 0)
sketch "スケッチ7" plane through (0, 0, 0) normal (0, 0, -1) x (-1, 0, 0)
  circle A0 centre (139.5445, -10.0968) radius 1.25 projected
  circle A1 centre (105.5257, -16.4118) radius 7.025 projected
  circle A2 centre (72.8083, -2.3784) radius 1.5 projected
  circle A3 centre (79.2726, -40.4563) radius 1.5 projected
  circle A4 centre (145.5257, 0.5882) radius 1.5 projected
  circle A5 centre (65.5257, -10.4118) radius 1.5 projected
  circle A6 centre (75.5257, 23.124) radius 1.5 projected
  circle A7 centre (122.6945, 30.2622) radius 1.5 projected
  line L0 (149.0922, 3.3323) -> (126.261, 33.0062) projected
  arc A8 (126.261, 33.0062) -> (122.0212, 34.7115) centre (122.6945, 30.2622) ccw projected
  line L1 (122.0212, 34.7115) -> (74.8523, 27.5733) projected
  arc A9 (74.8523, 27.5733) -> (71.2133, 24.4099) centre (75.5257, 23.124) ccw projected
  line L2 (71.2133, 24.4099) -> (61.2133, -9.1259) projected
  arc A10 (61.2133, -9.1259) -> (61.4337, -12.2841) centre (65.5257, -10.4118) ccw projected
  line L3 (61.4337, -12.2841) -> (75.1806, -42.3286) projected
  arc A11 (75.1806, -42.3286) -> (78.813, -44.9328) centre (79.2726, -40.4563) ccw projected
  line L4 (78.813, -44.9328) -> (102.3494, -47.3492) projected
  arc A12 (102.3494, -47.3492) -> (132.6633, -31.6026) centre (105.5257, -16.4118) ccw projected
  line L5 (132.6633, -31.6026) -> (149.4523, -1.6098) projected
  arc A13 (149.4523, -1.6098) -> (149.0922, 3.3323) centre (145.5257, 0.5882) ccw projected
  circle A14 centre (145.5257, 0.5882) radius 1.5
  arc A15 (128.1942, 33.7759) -> (117.8885, 25.8468) centre (145.5257, 0.5882) ccw construction
  arc A16 (127.4998, 35.1056) -> (116.7813, 26.8587) centre (145.5257, 0.5882) ccw
  arc A17 (128.8885, 32.4463) -> (118.9958, 24.8348) centre (145.5257, 0.5882) ccw
  arc A18 (128.8885, 32.4463) -> (127.4998, 35.1056) centre (128.1942, 33.7759) ccw
  arc A19 (116.7813, 26.8587) -> (118.9958, 24.8348) centre (117.8885, 25.8468) ccw
  line L6 (178.9476, 98.4754) -> (172.4962, -106.9557)
  circle A20 centre (145.5257, 0.5882) radius 4.5
  arc A21 (130.2772, 29.7871) -> (121.2102, 22.8109) centre (145.5257, 0.5882) ccw
  arc A22 (130.2772, 29.7871) -> (126.1111, 37.7648) centre (128.1942, 33.7759) ccw
  arc A23 (126.1111, 37.7648) -> (114.5668, 28.8826) centre (145.5257, 0.5882) ccw
  arc A24 (114.5668, 28.8826) -> (121.2102, 22.8109) centre (117.8885, 25.8468) ccw
  line L7 (127.5208, 38.2253) -> (174.213, 45.2914)
  arc A25 (123.2304, 25.7942) -> (125.7514, 26.9599) centre (122.6945, 30.2622) ccw projected
  line L8 (125.7514, 26.9599) -> (143.1172, 4.3894)
  arc A26 (143.1172, 4.3894) -> (141.0367, 0.9029) centre (145.5257, 0.5882) ccw projected
  line L9 (149.0922, 3.3323) -> (126.261, 33.0062) projected
  line L10 (174.213, 45.2914) -> (177.2058, 43.0125)
  line L11 (149.2108, -1.9944) -> (177.0395, 37.7154)
  line L12 (122.0212, 34.7115) -> (74.8523, 27.5733) projected
  point P0 (0, 0)
  point P1 (125.7643, 26.9431)
  point P2 (143.1172, 4.3894)
  point P3 (126.0168, 37.7154)
  point P4 (125.4386, 26.6957)
  point P5 (149.3413, -1.8082)
  dimension "d55" = 3
  dimension "d56" = 3
  dimension "d57" = 20
  dimension "d59" = 3
  dimension "d60" = 3
  dimension "d61" = 10
  constraints: 22 point on circle, 11 centre point, 10 end point, 6 tangent, 2 coincident, 2 parallel, 2 point on line, 4 other
  measures "d55" diameter of A14
  measures "d56" diameter of A18
  measures "d59" radial gap between concentric circles of A14 A20
  measures "d60" radial gap between concentric circles of A19 A24
ref_plane "作業平面1" through (0, 0, -3) normal (0, 0, -1) x (-1, 0, 0)
sketch "スケッチ8" plane through (0, 0, -3) normal (0, 0, -1) x (-1, 0, 0)
  line L0 (174.213, 45.2914) -> (127.5208, 38.2253) projected
  arc A0 (127.5208, 38.2253) -> (126.1111, 37.7648) centre (128.1942, 33.7759) ccw projected
  arc A1 (126.1111, 37.7648) -> (114.5668, 28.8826) centre (145.5257, 0.5882) ccw projected
  arc A2 (114.5668, 28.8826) -> (121.2102, 22.8109) centre (117.8885, 25.8468) ccw projected
  arc A3 (125.4386, 26.6957) -> (121.2102, 22.8109) centre (145.5257, 0.5882) ccw projected
  arc A4 (125.4386, 26.6957) -> (125.7514, 26.9599) centre (122.6945, 30.2622) ccw projected
  line L1 (125.7514, 26.9599) -> (143.1172, 4.3894) projected
  arc A5 (143.1172, 4.3894) -> (149.4523, -1.6098) centre (145.5257, 0.5882) ccw projected
  line L2 (149.4523, -1.6098) -> (149.3413, -1.8082) projected
  line L3 (149.3413, -1.8082) -> (177.0395, 37.7154) projected
  line L4 (177.0395, 37.7154) -> (177.2058, 43.0125) projected
  line L5 (177.2058, 43.0125) -> (174.213, 45.2914) projected
  circle A6 centre (145.5257, 0.5882) radius 1.5 projected
  arc A7 (116.7813, 26.8587) -> (118.9958, 24.8348) centre (117.8885, 25.8468) ccw projected
  arc A8 (127.4998, 35.1056) -> (116.7813, 26.8587) centre (145.5257, 0.5882) ccw projected
  arc A9 (128.8885, 32.4463) -> (127.4998, 35.1056) centre (128.1942, 33.7759) ccw projected
  arc A10 (128.8885, 32.4463) -> (118.9958, 24.8348) centre (145.5257, 0.5882) ccw projected
  line L6 (174.213, 45.2914) -> (127.5208, 38.2253) projected
  line L7 (177.0395, 37.7154) -> (177.2058, 43.0125) projected
  line L8 (149.3413, -1.8082) -> (177.0395, 37.7154) projected
  line L9 (125.7514, 26.9599) -> (143.1172, 4.3894) projected
  line L10 (127.5208, 38.2253) -> (136.18, 32.2797)
  line L11 (136.18, 32.2797) -> (140.4689, 37.7075)
  line L12 (140.4689, 37.7075) -> (146.1718, 33.7918)
  line L13 (146.1718, 33.7918) -> (150.4607, 39.2196)
  line L14 (150.4607, 39.2196) -> (156.1635, 35.3039)
  line L15 (156.1635, 35.3039) -> (160.4524, 40.7317)
  line L16 (160.4524, 40.7317) -> (166.1553, 36.816)
  line L17 (166.1553, 36.816) -> (170.4442, 42.2438)
  line L18 (136.18, 32.2797) -> (166.1553, 36.816) construction
  line L19 (170.4442, 42.2438) -> (177.0395, 37.7154)
  point P0 (0, 0)
  constraints: 20 end point, 8 parallel, 4 equal length, 2 point on line
equation "\"d41\" = d40"
